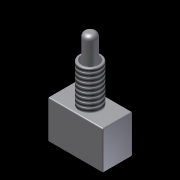
# Autodesk Inventor part: Schalter
Saved by Autodesk Inventor 2011 SP1 (Build 150282100, 282)
## iProperties
Created: 2012-07-12
Part Number: Schalter
Document SubType Name: Modeling
Designer: nfischer
Density: 1 g/cm^3
Author: nfischer
Autodesk Inventor part; units mm, degrees
ref_plane "YZ Plane" through (0, 0, 0) normal (1, 0, 0) x (0, 1, 0)
ref_plane "XZ Plane" through (0, 0, 0) normal (0, 1, 0) x (-1, 0, 0)
ref_plane "XY Plane" through (0, 0, 0) normal (0, 0, 1) x (1, 0, 0)
sketch "Skizze1" plane through (0, 0, 0) normal (0, 0, 1) x (1, 0, 0)
  line L0 (-6.35, 3.429) -> (6.35, 3.429)
  line L1 (6.35, 3.429) -> (6.35, -3.429)
  line L2 (6.35, -3.429) -> (-6.35, -3.429)
  line L3 (-6.35, -3.429) -> (-6.35, 3.429)
  point P0 (0, 0)
  point P1 (6.35, 0)
  point P2 (0, -3.429)
  dimension "d0" = 12.7
  dimension "d1" = 6.858
  constraints: 8 end point, 2 midpoint, 2 parallel, 1 horizontal, 1 horizontal alignment, 1 perpendicular, 1 vertical alignment
  measures "d0" distance of L1.end L2.end
  measures "d1" distance of L2.end L0.start
extrude "Extrusion1" add sketch "Skizze1" along normal blind 8.89
sketch "Skizze2" plane through (0, 0, 8.89) normal (0, 0, 1) x (1, 0, 0)
  circle A0 centre (0, 0) radius 2.5
  circle A1 centre (0, 0) radius 2.25
  dimension "d4" = 5
  dimension "d10" = 4.5
  constraints: 2 centre point, 2 coincident
  measures "d4" diameter of A0
  measures "d10" diameter of A1
extrude "Extrusion2" add sketch "Skizze2" along normal blind 8.89 contours A0 | A1
thread "Gewinde1" size "M6x1" class "6g" standard "ANSI Metric M Profile" full length
fillet "Rundung1" radius 0.25 1 edges at (-2.5, 0, 17.78)
sketch "Skizze3" plane through (0, 0, 17.78) normal (0, 0, 1) x (1, 0, 0)
  circle A0 centre (0, 0) radius 2.25 projected
  circle A1 centre (0, 0) radius 2
  dimension "d11" = 4
  constraints: 1 centre point, 1 coincident
  measures "d11" diameter of A1
extrude "Extrusion3" cut sketch "Skizze3" against normal blind 5 contours A1
sketch "Skizze4" plane through (0, 0, 12.78) normal (0, 0, 1) x (1, 0, 0)
  circle A0 centre (0, 0) radius 2 projected
  circle A1 centre (0, 0) radius 1.46
  dimension "d14" = 2.92
  constraints: 1 centre point, 1 coincident
  measures "d14" diameter of A1
extrude "Extrusion4" add sketch "Skizze4" along normal blind 10.67 contours A1
fillet "Rundung3" radius 0.25 12 edges at (0, 3.429, 8.89) (-6.35, 0, 8.89) (0, -3.429, 8.89) (6.35, 0, 8.89) (-6.35, 0, 0) (-6.35, -3.429, 4.445) (-6.35, 3.429, 4.445) (6.35, 3.429, 4.445) (0, 3.429, 0) (6.35, -3.429, 4.445) (0, -3.429, 0) (6.35, 0, 0)
fillet "Rundung5" radius 1 1 edges at (-1.46, 0, 23.45)
